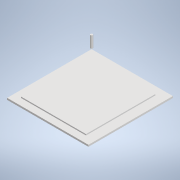
# Autodesk Inventor part: PCBBoard
Saved by Autodesk Inventor 2021 (Build 250183000, 183)
## iProperties
Created: 2020-12-14
Part Number: PCBBoard
Material: Generic
Document SubType Name: Modeling
Designer: soeren
Density: 1 g/cm^3
Appearance: Default
Author: soeren
Autodesk Inventor part; units mm, degrees
ref_plane "YZ Plane" through (0, 0, 0) normal (1, 0, 0) x (0, 1, 0)
ref_plane "XZ Plane" through (0, 0, 0) normal (0, 1, 0) x (-1, 0, 0)
ref_plane "XY Plane" through (0, 0, 0) normal (0, 0, 1) x (1, 0, 0)
sketch "Sketch1" plane through (0, 0, 0) normal (0, 1, 0) x (-1, 0, 0)
  line L0 (0, 0) -> (70.75, 0)
  line L1 (70.75, 0) -> (70.75, -73.5)
  line L2 (70.75, -73.5) -> (0, -73.5)
  line L3 (0, -73.5) -> (0, 0)
  dimension "d0" = 73.5
  dimension "d1" = 70.75
  constraints: 8 end point, 2 parallel, 1 horizontal, 1 perpendicular
  measures "d0" distance of L0.end L1.end
  measures "d1" distance of L1.end L2.end
extrude "Extrusion1" add sketch "Sketch1" along normal blind 1.5
sketch "Sketch2" plane through (0, 1.5, 0) normal (0, 1, 0) x (1, 0, 0)
  line L0 (-64.75, 6) -> (-8.1, 6)
  line L1 (-8.1, 6) -> (-8.1, 66.3)
  line L2 (-8.1, 66.3) -> (-64.75, 66.3)
  line L3 (-64.75, 66.3) -> (-64.75, 6)
  line L4 (0, 0) -> (0, 73.5) projected
  line L5 (0, 73.5) -> (-70.75, 73.5) projected
  line L6 (-70.75, 0) -> (0, 0) projected
  line L7 (-70.75, 73.5) -> (-70.75, 0) projected
  dimension "d4" = 8.1
  dimension "d5" = 7.2
  dimension "d6" = 6
  dimension "d7" = 6
  constraints: 8 end point, 2 parallel, 1 horizontal, 1 perpendicular
  measures "d4" distance between parallel lines of L1 L4
  measures "d5" distance between parallel lines of L5 L2
  measures "d6" distance between parallel lines of L6 L0
  measures "d7" distance between parallel lines of L7 L3
extrude "Extrusion2" add sketch "Sketch2" along normal blind 1 contours L3 L2 L1 L0
sketch "Sketch3" plane through (0, 2.5, 0) normal (0, 1, 0) x (1, 0, 0)
  line L0 (0, 73.5) -> (-70.75, 73.5) projected
  circle A0 centre (-70.75, 73.5) radius 1
  point P0 (0, 0)
  dimension "d10" = 2
  constraints: 1 centre point
  measures "d10" diameter of A0
extrude "Extrusion3" add sketch "Sketch3" along normal blind 10
body "Solid1"
